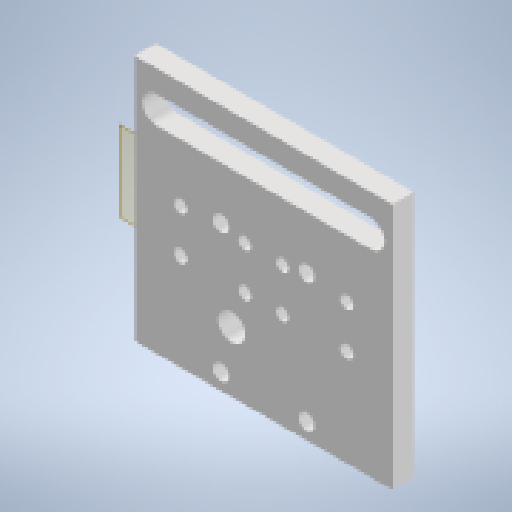
# Autodesk Inventor part: деталь на которой рельсы
Saved by Autodesk Inventor 2024.2 (Build 282272000, 272)
## iProperties
Created: 2025-11-27
Part Number: деталь на которой рельсы
Material: Типовые
Document SubType Name: Modeling
Designer: katya_notebook
Density: 1 g/cm^3
Appearance: По умолчанию
Author: katya_notebook
Autodesk Inventor part; units mm, degrees
ref_plane "YZ Plane" through (0, 0, 0) normal (1, 0, 0) x (0, 1, 0)
ref_plane "XZ Plane" through (0, 0, 0) normal (0, 1, 0) x (-1, 0, 0)
ref_plane "XY Plane" through (0, 0, 0) normal (0, 0, 1) x (1, 0, 0)
ref_plane "РабПлоскость1" through (30.6718, 18.7359, -492.3) normal (0, 0, 1) x (1, 0, 0)
sketch "Эскиз1" plane through (30.6718, 18.7359, -492.3) normal (0, 0, 1) x (1, 0, 0)
  line L0 (9.0963, 0) -> (4.4963, 0) projected
  line L1 (4.4963, 0) -> (4.4963, -13.5) projected
  line L2 (9.0963, -13.5) -> (4.4963, -13.5) projected
  line L3 (9.0963, -13.5) -> (9.0963, 0) projected
  circle A0 centre (6.7963, -2.75) radius 1.2 projected
  circle A1 centre (6.7963, -10.75) radius 1.2 projected
  line L4 (21.0963, 0) -> (16.4963, 0) projected
  line L5 (16.4963, 0) -> (16.4963, -13.5) projected
  line L6 (21.0963, -13.5) -> (16.4963, -13.5) projected
  line L7 (21.0963, -13.5) -> (21.0963, 0) projected
  circle A2 centre (18.7963, -2.75) radius 1.2 projected
  circle A3 centre (18.7963, -10.75) radius 1.2 projected
  line L8 (28.0963, 0) -> (23.4963, 0) projected
  line L9 (23.4963, 0) -> (23.4963, -13.5) projected
  line L10 (28.0963, -13.5) -> (23.4963, -13.5) projected
  line L11 (28.0963, -13.5) -> (28.0963, 0) projected
  circle A4 centre (25.7963, -2.75) radius 1.2 projected
  circle A5 centre (25.7963, -10.75) radius 1.2 projected
  line L12 (40.0963, 0) -> (35.4963, 0) projected
  line L13 (35.4963, 0) -> (35.4963, -13.5) projected
  line L14 (40.0963, -13.5) -> (35.4963, -13.5) projected
  line L15 (40.0963, -13.5) -> (40.0963, 0) projected
  circle A6 centre (37.7963, -2.75) radius 1.2 projected
  circle A7 centre (37.7963, -10.75) radius 1.2 projected
  circle A8 centre (36.2999, 10.4999) radius 2.5 projected
  circle A9 centre (36.2999, 10.4999) radius 1 projected
  circle A10 centre (16.3, -17.5) radius 2.5 projected
  circle A11 centre (16.3, -17.5) radius 1 projected
  line L16 (-2.7279, 21.2173) -> (47.2721, 21.2173)
  line L17 (47.2721, 21.2173) -> (47.2721, -28.7827)
  line L18 (47.2721, -28.7827) -> (-2.7279, -28.7827)
  line L19 (-2.7279, -28.7827) -> (-2.7279, 21.2173)
  line L20 (22.2721, -16.5) -> (22.2721, -5.5248)
  line L21 (13.8, -23.7827) -> (31.824, -23.7827)
  line L22 (2.2721, 13.0833) -> (42.2721, 13.0833)
  line L23 (2.2721, 7.9833) -> (42.2721, 7.9833)
  circle A12 centre (2.2721, 10.5333) radius 2.55
  circle A13 centre (42.2721, 10.5333) radius 2.55
  point P0 (-30.6718, -18.7359)
  point P1 (-2.7279, -3.7827)
  point P2 (42.2721, 13.0833)
  dimension "d0" = 50
  dimension "d1" = 50
  dimension "d2" = 25
  dimension "d3" = 5
  dimension "d10" = 40
  dimension "d11" = 5
  dimension "d13" = 5
  dimension "d14" = 5.1
  constraints: 16 end point, 5 horizontal, 2 parallel, 2 point on circle, 2 vertical, 1 centre point, 1 midpoint, 1 perpendicular, 3 other
  measures "d0" distance of L16.end L17.end
  measures "d1" distance of L16.start L16.end
  measures "d2" distance from line of point (-2.728, -3.783) L20
  measures "d3" distance between parallel lines of L18 L21
  measures "d10" distance of L22.start L22.end
  measures "d11" distance from line of L19 L22.start
  measures "d13" distance from line of L19 L23.start
  measures "d14" diameter of A12
extrude "Выдавливание1" add sketch "Эскиз1" along normal blind 4 contours L3 L2 L1 L0 | L7 L6 L5 L4 | L11 L10 L9 L8 | L15 L14 L13 L12 | L16 L17 L18 L19
sketch "Эскиз2" plane through (30.6718, 18.7359, -488.3) normal (0, 0, 1) x (1, 0, 0)
  circle A0 centre (30.2221, -1.7827) radius 1.5 projected
  circle A1 centre (14.3221, -1.7827) radius 1.5 projected
  circle A2 centre (30.2221, -25.7827) radius 1.5 projected
  circle A3 centre (14.3221, -25.7827) radius 1.5 projected
  point P0 (-30.6718, -18.7359)
extrude "Выдавливание2" cut sketch "Эскиз2" against normal blind 10
sketch "Эскиз3" plane through (30.6718, 18.7359, -488.3) normal (0, 0, 1) x (1, 0, 0)
  line L0 (47.2721, 21.2173) -> (-2.7279, 21.2173) projected
  line L1 (47.2721, -28.7827) -> (47.2721, 21.2173) projected
  line L2 (-2.7279, 21.2173) -> (47.2721, 21.2173)
  line L3 (47.2721, 21.2173) -> (47.2721, 17.2173)
  line L4 (47.2721, 17.2173) -> (-2.7279, 17.2173)
  line L5 (-2.7279, 17.2173) -> (-2.7279, 21.2173)
  point P0 (-30.6718, -18.7359)
  dimension "d15" = 4
  constraints: 8 end point, 2 parallel, 1 horizontal, 1 perpendicular, 1 point on line
  measures "d15" distance of L0.start L3.end
extrude "Выдавливание3" cut sketch "Эскиз3" against normal blind 10
sketch "Эскиз4" plane through (30.6718, 18.7359, -488.3) normal (0, 0, 1) x (1, 0, 0)
  line L0 (-2.7279, 17.2173) -> (-2.7279, -28.7827) projected
  line L1 (47.2721, 17.2173) -> (-2.7279, 17.2173) projected
  line L2 (-2.7279, -28.7827) -> (-1.7279, -28.7827)
  line L3 (-1.7279, -28.7827) -> (-1.7279, 17.2173)
  line L4 (-1.7279, 17.2173) -> (-2.7279, 17.2173)
  line L5 (-2.7279, 17.2173) -> (-2.7279, -28.7827)
  line L6 (47.2721, -28.7827) -> (47.2721, 17.2173) projected
  line L7 (-2.7279, -28.7827) -> (47.2721, -28.7827) projected
  line L8 (47.2721, 17.2173) -> (46.2721, 17.2173)
  line L9 (46.2721, 17.2173) -> (46.2721, -28.7827)
  line L10 (46.2721, -28.7827) -> (47.2721, -28.7827)
  line L11 (47.2721, -28.7827) -> (47.2721, 17.2173)
  point P0 (-30.6718, -18.7359)
  dimension "d18" = 1
  dimension "d19" = 1
  constraints: 16 end point, 4 parallel, 2 horizontal, 2 perpendicular, 2 point on line
  measures "d18" distance of L0.end L2.end
  measures "d19" distance of L6.start L9.end
extrude "Выдавливание4" cut sketch "Эскиз4" against normal blind 10 contours L1 L3 L2 L0 | L1 L6 L7 L9
